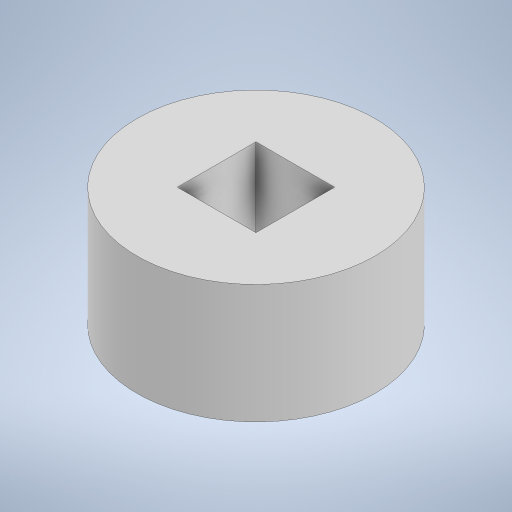
# Autodesk Inventor part: 111
Saved by Autodesk Inventor 2023 (Build 270158000, 158)
## iProperties
Created: 2024-11-14
Part Number: 111
Material: Generic
Document SubType Name: Sheet Metal
Designer: 1ZHUSAM
Density: 1 g/cm^3
Sheet Metal Rule: Default_mm
Appearance: Default
Author: 1ZHUSAM
Autodesk Inventor part; units mm, degrees
ref_plane "YZ Plane" through (0, 0, 0) normal (1, 0, 0) x (0, 1, 0)
ref_plane "XZ Plane" through (0, 0, 0) normal (0, 1, 0) x (-1, 0, 0)
ref_plane "XY Plane" through (0, 0, 0) normal (0, 0, 1) x (1, 0, 0)
sketch "Sketch1" plane through (0, 0, 0) normal (0, 1, 0) x (-1, 0, 0)
  circle A0 centre (0, 0) radius 5
  line L0 (1.651, 1.651) -> (-1.651, 1.651)
  line L1 (-1.651, 1.651) -> (-1.651, -1.651)
  line L2 (-1.651, -1.651) -> (1.651, -1.651)
  line L3 (1.651, -1.651) -> (1.651, 1.651)
  line L4 (1.651, 1.651) -> (-1.651, -1.651) construction
  line L5 (-1.651, 1.651) -> (1.651, -1.651) construction
  dimension "d0" = 10
  dimension "d1" = 3.302
  dimension "d2" = 3.302
  constraints: 12 end point, 2 midpoint, 2 parallel, 1 centre point, 1 coincident, 1 horizontal, 1 perpendicular
  measures "d0" diameter of A0
  measures "d1" distance of L2.end L1.end
  measures "d2" distance of L1.end L0.end
extrude "Extrusion1" add sketch "Sketch1" along normal blind 5
equation "\"BendRadius\" = Thickness"
equation "\"BendReliefWidth\" = Thickness"
equation "\"BendReliefDepth\" = 0.5 * Thickness"
equation "\"CornerReliefSize\" = 4 * Thickness"
equation "\"MinimumRemnant\" = 2 * Thickness"
equation "\"TransitionRadius\" = BendRadius"
equation "\"JacobiRadiusSize\" = BendRadius"
equation "\"GapSize\" = Thickness"
equation "\"Thickness\" = 0.5"
body "Solid1"
